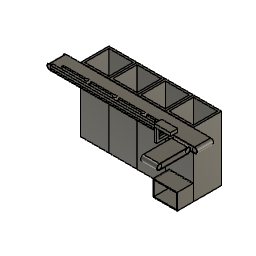
e-waste (Autodesk Fusion 360 design; units mm, degrees)
Autodesk Fusion 360 part; units mm, degrees
sketch "Sketch1" plane through (0, 0, 0) normal (0, 0, 1) x (1, 0, 0)
sketch "Sketch1 (2)" plane through (0, 0, 0) normal (0, 0, 1) x (1, 0, 0) in component "bin"
sketch "Sketch2" plane through (0, 0, 0) normal (0, 0, 1) x (1, 0, 0) in component "bin"
sketch "Sketch3" plane through (0, 0, 0) normal (0, 0, 1) x (1, 0, 0) in component "bin"
sketch "Sketch4" plane through (0, 0, 0) normal (0, 0, 1) x (1, 0, 0) in component "bin"
  line L0 (0, 0) -> (350, 0)
  line L1 (350, 0) -> (350, 350)
  line L2 (350, 350) -> (0, 350)
  line L3 (0, 350) -> (0, 0)
  dimension "d2" = 350
  dimension "d3" = 350
  constraint coincident L0.start L3.end
  constraint horizontal L0
  constraint perpendicular L0 L1
  constraint perpendicular L1 L2
  constraint perpendicular L0 L3
  measures "d2" distance of L0.start L0.end
  measures "d3" distance of L0.end L1.end
sketch "Sketch5" plane through (0, 0, 0) normal (0, 0, 1) x (1, 0, 0) in component "bin"
extrude "Extrude1" add sketch "Sketch4" along normal blind 800 makes body 1 in component "bin"
sketch "Sketch6" plane through (0, 0, 800) normal (0, 0, 1) x (-1, 0, 0) in component "bin"
  line L0 (0, -350) -> (0, 0)
  line L1 (0, 0) -> (-350, 0)
  line L2 (-350, 0) -> (-350, -350)
  line L3 (-350, -350) -> (0, -350)
  line L4 (-25, -325) -> (-325, -325)
  line L5 (-325, -325) -> (-325, -25)
  line L6 (-325, -25) -> (-25, -25)
  line L7 (-25, -25) -> (-25, -325)
  constraint perpendicular L0 L4
  constraint perpendicular L4 L5
  constraint perpendicular L5 L6
  constraint perpendicular L4 L7
extrude "Extrude2" cut sketch "Sketch6" against normal blind 775 contours L4 L5 L6 L7 bodies 1 in component "bin"
sketch "Sketch1 (3)" plane through (0, 0, 0) normal (0, 0, 1) x (1, 0, 0) in component "paddle"
  circle A0 centre (1000, 0) radius 20
  dimension "d9" = 40
  measures "d9" diameter of A0
extrude "Extrude1'" add sketch "Sketch1 (3)" along normal blind 50 separate body makes body 2 in component "paddle"
sketch "Sketch2 (2)" plane through (0, 0, 0) normal (0, 0, 1) x (1, 0, 0) in component "paddle"
  line L0 (1000, 0) -> (1000, 10)
  line L1 (1000, 10) -> (700, 10)
  line L2 (700, 10) -> (700, 0)
  line L3 (700, 0) -> (1000, 0)
  line L4 (700, 0) -> (700, -10)
  line L5 (700, -10) -> (1000, -10)
  line L6 (1000, -10) -> (1000, 0)
  line L7 (1000, 0) -> (700, 0)
  constraint perpendicular L0 L1
  constraint parallel L0 L2
  constraint parallel L1 L3
  constraint vertical L0
  constraint perpendicular L4 L5
  constraint parallel L4 L6
  constraint parallel L5 L7
  constraint perpendicular L3 L4
extrude "Extrude2'" add sketch "Sketch2 (2)" along normal blind 50 bodies 2 in component "paddle"
sketch "Sketch1 (4)" plane through (0, 0, 0) normal (0, 0, 1) x (1, 0, 0) in component "belt sensor"
  line L0 (1400, -450) -> (1200, -450)
  line L1 (1200, -450) -> (1200, -800)
  line L2 (1200, -800) -> (1400, -800)
  line L3 (1400, -800) -> (1400, -450)
  constraint horizontal L0
  constraint perpendicular L0 L1
  constraint perpendicular L1 L2
  constraint perpendicular L0 L3
extrude "Extrude1''" add sketch "Sketch1 (4)" along normal blind 70 separate body makes body 3 in component "belt sensor"
sketch "Sketch2 (3)" plane through (1400, 0, 0) normal (1, 0, 0) x (0, 1, 0) in component "belt sensor"
sketch "Sketch3 (2)" plane through (1400, 0, 0) normal (1, 0, 0) x (0, 1, 0) in component "belt sensor"
sketch "Sketch4 (2)" plane through (1400, 0, 0) normal (1, 0, 0) x (0, 1, 0) in component "belt sensor"
  circle A0 centre (-800, 35) radius 35
  circle A1 centre (-800, 35) radius 30
  constraint concentric A0 A1
extrude "Extrude2''" add sketch "Sketch4 (2)" against normal blind 200 bodies 3 in component "belt sensor"
sketch "Sketch5 (2)" plane through (1400, 0, 0) normal (1, 0, 0) x (0, 1, 0) in component "belt sensor"
  circle A0 centre (-450, 35) radius 35
  circle A1 centre (-450, 35) radius 30
  constraint concentric A0 A1
extrude "Extrude3" add sketch "Sketch5 (2)" against normal blind 200 bodies 3 in component "belt sensor"
sketch "Sketch6 (2)" plane through (1400, 0, 0) normal (1, 0, 0) x (0, 1, 0) in component "belt sensor"
  line L0 (-800, 65) -> (-450, 65)
  line L1 (-450, 65) -> (-450, 5)
  line L2 (-450, 5) -> (-800, 5)
  line L3 (-800, 5) -> (-800, 65)
  constraint horizontal L0
  constraint vertical L1
  constraint horizontal L2
  constraint vertical L3
extrude "Extrude4" cut sketch "Sketch6 (2)" against normal blind 300 bodies 3 in component "belt sensor"
sketch "Sketch7" plane through (1400, 0, 0) normal (1, 0, 0) x (0, 1, 0) in component "belt sensor"
  line L0 (-450, 5) -> (-800, 5)
  arc A0 (-800, 65) -> (-800, 5) centre (-800, 35) ccw
  line L1 (-800, 65) -> (-450, 65)
  arc A1 (-450, 5) -> (-450, 65) centre (-450, 35) ccw
  arc A2 (-450, 0) -> (-450, 70) centre (-450, 35) ccw
  line L2 (-450, 70) -> (-800, 70)
  arc A3 (-800, 70) -> (-800, 0) centre (-800, 35) ccw
  line L3 (-800, 0) -> (-450, 0)
  circle A4 centre (-800, 35) radius 27.5
  dimension "d42" = 55
  constraint concentric A0 A4
  measures "d42" diameter of A4
extrude "Extrude5" add sketch "Sketch7" against normal blind 200 separate body contours A4 makes body 4 in component "belt sensor"
sketch "Sketch8" plane through (1400, 0, 0) normal (1, 0, 0) x (0, 1, 0) in component "belt sensor"
  circle A0 centre (-800, 35) radius 27.5
  circle A1 centre (-450, 35) radius 27.5
  dimension "d45" = 55
  measures "d45" diameter of A1
extrude "Extrude6" add sketch "Sketch8" against normal blind 200 separate body contours A1 makes body 5 in component "belt sensor"
sketch "Sketch1 (5)" plane through (0, 0, 0) normal (0, 1, 0) x (1, 0, 0) in component "sensor"
  line L0 (0, -1000) -> (1500, -1000)
  line L1 (1500, -1000) -> (1500, -1250)
  line L2 (1500, -1250) -> (1470, -1250)
  line L3 (0, -1000) -> (0, -1030)
  line L4 (1470, -1250) -> (1470, -1030)
  line L5 (0, -1030) -> (1470, -1030)
  dimension "d48" = 1500
  dimension "d49" = 250
  dimension "d50" = 30
  dimension "d51" = 30
  dimension "d52" = 220
  constraint horizontal L0
  constraint perpendicular L0 L1
  constraint perpendicular L1 L2
  constraint perpendicular L0 L3
  constraint perpendicular L0 L4
  measures "d48" distance of L0.start L0.end
  measures "d49" distance of L0.end L1.end
  measures "d50" distance of L1.end L2.end
  measures "d51" distance of L0.start L3.end
  measures "d52" distance of L2.end L4.end
extrude "Extrude1'''" add sketch "Sketch1 (5)" along normal blind 30 separate body makes body 6 in component "sensor"
sketch "Sketch2 (4)" plane through (0, 0, 0) normal (0, -1, 0) x (1, 0, 0) in component "sensor"
sketch "Sketch3 (3)" plane through (1500, 0, 0) normal (1, 0, 0) x (0, 1, 0) in component "sensor"
  line L0 (0, 1250) -> (0, 1000)
  line L1 (0, 1000) -> (30, 1000)
  line L2 (30, 1000) -> (30, 1250)
  line L3 (30, 1250) -> (0, 1250)
  line L4 (60, 1250) -> (-30, 1250)
  line L5 (-30, 1250) -> (-30, 1210)
  line L6 (-30, 1210) -> (60, 1210)
  line L7 (60, 1210) -> (60, 1250)
  constraint horizontal L4
  constraint vertical L5
  constraint horizontal L6
  constraint vertical L7
extrude "Extrude2'''" add sketch "Sketch3 (3)" along normal blind 200 separate body contours L0 L2 L3 L4 L6 | L0 L4 L5 L6 | L2 L4 L6 L7 makes body 7 in component "sensor"
sketch "Sketch4 (3)" plane through (0, 0, 0) normal (0, -1, 0) x (1, 0, 0) in component "sensor"
sketch "Sketch5 (3)" plane through (0, 0, 0) normal (0, -1, 0) x (1, 0, 0) in component "sensor"
  line L0 (1500, 1000) -> (1470, 1000)
  line L1 (1470, 1000) -> (1470, 1250)
  line L2 (1470, 1250) -> (1500, 1250)
  line L3 (1500, 1250) -> (1500, 1000)
  constraint horizontal L0
  constraint vertical L1
  constraint horizontal L2
  constraint vertical L3
extrude "Extrude3'" cut sketch "Sketch5 (3)" against normal blind 500 bodies 6 in component "sensor"
sketch "Sketch6 (3)" plane through (0, 0, 0) normal (0, -1, 0) x (1, 0, 0) in component "sensor"
sketch "Sketch7 (2)" plane through (0, 0, 1030) normal (0, 0, 1) x (-1, 0, 0) in component "sensor"
  line L0 (0, 0) -> (-1470, 0)
  line L1 (-1470, 0) -> (-1470, -30)
  line L2 (-1470, -30) -> (0, -30)
  line L3 (0, -30) -> (0, 0)
  line L4 (-1470, 0) -> (-1470, 150)
  line L5 (-1470, 150) -> (-1440, 150)
  line L6 (-1440, 150) -> (-1440, 0)
  constraint coincident L0.end L1.start
  constraint perpendicular L0 L4
  constraint perpendicular L4 L5
  constraint coincident L0 L6.end
  constraint perpendicular L0 L6
extrude "Extrude4'" add sketch "Sketch7 (2)" against normal blind 30 contours L0 L4 L5 L6 bodies 6 in component "sensor"
sketch "Sketch8 (2)" plane through (0, 0, 1030) normal (0, 0, 1) x (-1, 0, 0) in component "sensor"
  line L0 (0, 0) -> (-1440, 0)
  line L1 (-1440, 0) -> (-1440, 150)
  line L2 (-1440, 150) -> (-1470, 150)
  line L3 (-1470, 150) -> (-1470, -30)
  line L4 (-1470, -30) -> (0, -30)
  line L5 (0, -30) -> (0, 0)
  line L6 (-1470, 150) -> (-1440, 150)
  line L7 (-1440, 150) -> (-1440, 120)
  line L8 (-1440, 120) -> (-1470, 120)
  line L9 (-1470, 120) -> (-1470, 150)
  constraint horizontal L6
  constraint vertical L7
  constraint horizontal L8
  constraint vertical L9
  constraint coincident L1 L7.end
  constraint coincident L2.end L3.start
extrude "Extrude5'" add sketch "Sketch8 (2)" along normal blind 200 contours L1 L2 L3 L6 L7 L8 L9 bodies 6 in component "sensor"
move_body "Move1" bodies 7 to x (1, 0, 0) y (0, 1, 0) z (0, 0, 1) at (-30, -150, 0) in component "sensor"
sketch "Sketch9" plane through (0, 0, 1210) normal (0, 0, -1) x (1, 0, 0) in component "sensor"
  line L0 (1470, 180) -> (1470, 90)
  line L1 (1470, 90) -> (1670, 90)
  line L2 (1670, 90) -> (1670, 180)
  line L3 (1670, 180) -> (1470, 180)
  line L4 (1470, 180) -> (1570, 180)
  line L5 (1570, 180) -> (1570, 90)
  circle A0 centre (1570, 135) radius 15
  dimension "d63" = 30
  constraint coincident L0.start L3.end
  constraint midpoint L3 L4.end
  constraint midpoint L1 L5.end
  constraint midpoint L5 A0.centre
  measures "d63" diameter of A0
extrude "Extrude6'" add sketch "Sketch9" along normal blind 20 contours L5 A0 | L5 A0 bodies 7 in component "sensor"
sphere "SpherePrimitive1" cut diameter 30 placed x (1, 0, 0) y (0, -1, 0) z (0, 0, -1) at (1570, -135, 1190) bodies 7 in component "sensor"
sphere "SpherePrimitive2" add diameter 30 placed x (1, 0, 0) y (0, 0, -1) z (0, 1, 0) at (1570, 0, 1190) separate body makes body 8 in component "sensor"
move_body "Move2" bodies 8 to x (1, 0, 0) y (0, 1, 0) z (0, 0, 1) at (0, -135, 0) in component "sensor"
move_body "Move1'" bodies 4 5 3 to x (1, 0, 0) y (0, 1, 0) z (0, 0, 1) at (0, 180, 750) in component "belt sensor"
move_body "Move3" bodies 6 to x (1, 0, 0) y (0, 1, 0) z (0, 0, 1) at (-300, -300, -150) in component "sensor"
move_body "Move4" bodies 7 8 to x (1, 0, 0) y (0, 1, 0) z (0, 0, 1) at (-300, -300, -170) in component "sensor"
move_body "Move1''" bodies 2 to x (1, 0, 0) y (0, 1, 0) z (0, 0, 1) at (0, -250, 850) in component "paddle"
move_body "Move5" bodies 6 7 8 to x (1, 0, 0) y (0, 1, 0) z (0, 0, 1) at (50, 0, 0) in component "sensor"
move_body "Move2'" bodies 2 to x (1, 0, 0) y (0, 1, 0) z (0, 0, 1) at (200, 0, 0) in component "paddle"
move_body "Move3'" bodies 2 to x (1, 0, 0) y (0, 1, 0) z (0, 0, 1) at (175, 0, 0) in component "paddle"
move_body "Move6" bodies 6 7 8 to x (1, 0, 0) y (0, 1, 0) z (0, 0, 1) at (175, 0, 0) in component "sensor"
move_body "Move2''" bodies 4 5 3 to x (1, 0, 0) y (0, 1, 0) z (0, 0, 1) at (200, 0, 0) in component "belt sensor"
sketch "Sketch1 (6)" plane through (0, 0, 0) normal (0, 1, 0) x (1, 0, 0) in component "belt"
  line L0 (0, 500) -> (1800, 500)
  line L1 (1800, 500) -> (1800, 430)
  line L2 (1800, 430) -> (0, 430)
  line L3 (0, 430) -> (0, 500)
  dimension "d68" = 1800
  dimension "d69" = 70
  constraint horizontal L0
  constraint perpendicular L0 L1
  constraint perpendicular L1 L2
  constraint perpendicular L0 L3
  measures "d68" distance of L0.start L0.end
  measures "d69" distance of L0.end L1.end
extrude "Extrude1''''" add sketch "Sketch1 (6)" along normal blind 200 separate body makes body 9 in component "belt"
sketch "Sketch2 (5)" plane through (0, 0, 0) normal (0, -1, 0) x (1, 0, 0) in component "belt"
  line L0 (1800, -430) -> (0, -430)
  line L1 (0, -430) -> (0, -500)
  line L2 (0, -500) -> (1800, -500)
  line L3 (1800, -500) -> (1800, -430)
  circle A0 centre (0, -465) radius 35
  circle A1 centre (0, -465) radius 30
  dimension "d72" = 60
  constraint midpoint L1 A0.centre
  constraint coincident L0.end A0
  constraint concentric A0 A1
  measures "d72" diameter of A1
extrude "Extrude2''''" add sketch "Sketch2 (5)" against normal blind 200 contours L1 A0 A1 picked at (-12.8396, -434.3307) bodies 9 in component "belt"
sketch "Sketch3 (4)" plane through (0, 0, 0) normal (0, -1, 0) x (1, 0, 0) in component "belt"
  line L0 (0, -500) -> (1800, -500)
  line L1 (1800, -500) -> (1800, -430)
  line L2 (1800, -430) -> (0, -430)
  arc A0 (0, -430) -> (0, -500) centre (0, -465) ccw
  arc A1 (0, -435) -> (0, -495) centre (0, -465) ccw
  line L3 (0, -435) -> (0, -495)
  circle A2 centre (1800, -465) radius 35
  circle A3 centre (1800, -465) radius 30
  dimension "d75" = 60
  constraint midpoint L1 A2.centre
  constraint coincident L1.end A2
  constraint concentric A2 A3
  measures "d75" diameter of A3
extrude "Extrude3''" add sketch "Sketch3 (4)" against normal blind 200 contours L1 A2 A3 picked at (1831.4014, -454.0493) bodies 9 in component "belt"
sketch "Sketch4 (4)" plane through (0, 0, 0) normal (0, -1, 0) x (1, 0, 0) in component "belt"
  line L0 (1800, -430) -> (0, -430)
  arc A0 (0, -430) -> (0, -500) centre (0, -465) ccw
  line L1 (0, -500) -> (1800, -500)
  arc A1 (1800, -500) -> (1800, -430) centre (1800, -465) ccw
  arc A2 (1800, -495) -> (1800, -435) centre (1800, -465) ccw
  line L2 (1800, -495) -> (1800, -435)
  arc A3 (0, -435) -> (0, -495) centre (0, -465) ccw
  line L3 (0, -435) -> (0, -495)
  line L4 (0, -435) -> (1800, -435)
  line L5 (1800, -435) -> (1800, -495)
  line L6 (1800, -495) -> (0, -495)
  line L7 (0, -495) -> (0, -435)
  constraint horizontal L4
  constraint vertical L5
  constraint horizontal L6
  constraint vertical L7
  constraint coincident A2.start L2.start
  constraint coincident A3.start L3.start
extrude "Extrude4''" cut sketch "Sketch4 (4)" against normal blind 300 contours L2 L3 L4 L5 L6 L7 bodies 9 in component "belt"
sketch "Sketch5 (4)" plane through (0, 0, 0) normal (0, -1, 0) x (1, 0, 0) in component "belt"
  line L0 (0, -435) -> (1800, -435)
  arc A0 (1800, -495) -> (1800, -435) centre (1800, -465) ccw
  line L1 (1800, -495) -> (0, -495)
  arc A1 (0, -435) -> (0, -495) centre (0, -465) ccw
  line L2 (1800, -430) -> (0, -430)
  arc A2 (0, -430) -> (0, -500) centre (0, -465) ccw
  line L3 (0, -500) -> (1800, -500)
  arc A3 (1800, -500) -> (1800, -430) centre (1800, -465) ccw
  circle A4 centre (0, -465) radius 27.5
  circle A5 centre (1800, -465) radius 27.5
  dimension "d80" = 55
  dimension "d81" = 55
  constraint concentric A1 A4
  constraint concentric A0 A5
  measures "d80" diameter of A4
  measures "d81" diameter of A5
extrude "Extrude5''" add sketch "Sketch5 (4)" against normal blind 200 separate body contours A4 | A5 makes body 10 at (27.3633, 66.6667, -467.7381) makes body 11 at (1816.053, 133.3333, -442.6717) in component "belt"
move_body "Move1'''" bodies 10 9 11 to x (1, 0, 0) y (0, 1, 0) z (0, 0, 1) at (0, -225, 1250) in component "belt"
move_body "Move2'''" bodies 10 9 11 to x (1, 0, 0) y (0, 1, 0) z (0, 0, 1) at (-160, 0, 0) in component "belt"
sketch "Sketch1 (7)" plane through (0, 0, 0) normal (0, 1, 0) x (1, 0, 0) in component "power"
  line L0 (1400, 0) -> (1100, 0)
  line L1 (1100, 0) -> (1100, -200)
  line L2 (1100, -200) -> (1400, -200)
  line L3 (1400, -200) -> (1400, 0)
  constraint horizontal L0
  constraint perpendicular L0 L1
  constraint perpendicular L1 L2
  constraint perpendicular L0 L3
extrude "Extrude1'''''" add sketch "Sketch1 (7)" against normal blind 200 separate body makes body 12 in component "power"
sketch "Sketch2 (6)" plane through (0, -200, 0) normal (0, -1, 0) x (1, 0, 0) in component "power"
  line L0 (1400, 0) -> (1400, 200)
  line L1 (1400, 200) -> (1100, 200)
  line L2 (1100, 200) -> (1100, 0)
  line L3 (1100, 0) -> (1400, 0)
  line L4 (1110, 190) -> (1390, 190)
  line L5 (1390, 190) -> (1390, 10)
  line L6 (1390, 10) -> (1110, 10)
  line L7 (1110, 10) -> (1110, 190)
  constraint perpendicular L0 L4
  constraint perpendicular L4 L5
  constraint perpendicular L5 L6
  constraint perpendicular L4 L7
extrude "Extrude2'''''" cut sketch "Sketch2 (6)" against normal blind 190 contours L4 L5 L6 L7 bodies 12 in component "power"
sketch "Sketch2 (7)" plane through (0, 0, 0) normal (0, 0, 1) x (1, 0, 0)
sketch "Sketch1 (8)" plane through (0, 0, 0) normal (0, 0, 1) x (1, 0, 0) in component "vibrator"
  line L0 (0, 850) -> (200, 850)
  line L1 (200, 850) -> (200, 1050)
  line L2 (200, 1050) -> (0, 1050)
  line L3 (0, 1050) -> (0, 850)
  dimension "d89" = 200
  dimension "d90" = 200
  constraint horizontal L0
  constraint perpendicular L0 L1
  constraint perpendicular L1 L2
  constraint perpendicular L0 L3
  measures "d89" distance of L0.start L0.end
  measures "d90" distance of L0.end L1.end
extrude "Extrude1''''''" add sketch "Sketch1 (8)" along normal blind 15 separate body makes body 13 in component "vibrator"
move_body "Move1''''" bodies 13 to x (1, 0, 0) y (0, 1, 0) z (0, 0, 1) at (75, -775, 300) in component "vibrator"
component "bin" placed x (1, 0, 0) y (0, 1, 0) z (0, 0, 1) at (0, 0, 0)
component "paddle" placed x (1, 0, 0) y (0, 1, 0) z (0, 0, 1) at (0, 0, 0)
component "belt sensor" placed x (1, 0, 0) y (0, 1, 0) z (0, 0, 1) at (0, 0, 0)
component "sensor" placed x (1, 0, 0) y (0, 1, 0) z (0, 0, 1) at (0, 0, 0)
component "bin" placed x (1, 0, 0) y (0, 1, 0) z (0, 0, 1) at (350, 0, 0)
component "bin" placed x (1, 0, 0) y (0, 1, 0) z (0, 0, 1) at (700, 0, 0)
component "bin" placed x (1, 0, 0) y (0, 1, 0) z (0, 0, 1) at (1050, 0, 0)
component "belt" placed x (1, 0, 0) y (0, 1, 0) z (0, 0, 1) at (0, 0, 0)
component "paddle" placed x (1, 0, 0) y (0, 1, 0) z (0, 0, 1) at (-350, 0, 0)
component "paddle" placed x (1, 0, 0) y (0, 1, 0) z (0, 0, 1) at (-700, 0, 0)
component "paddle" placed x (1, 0, 0) y (0, 1, 0) z (0, 0, 1) at (0, 0, 0)
component "power" placed x (1, 0, 0) y (0, 1, 0) z (0, 0, 1) at (0, 0, 0)
component "vibrator" placed x (1, 0, 0) y (0, 1, 0) z (0, 0, 1) at (0, 0, 0)
